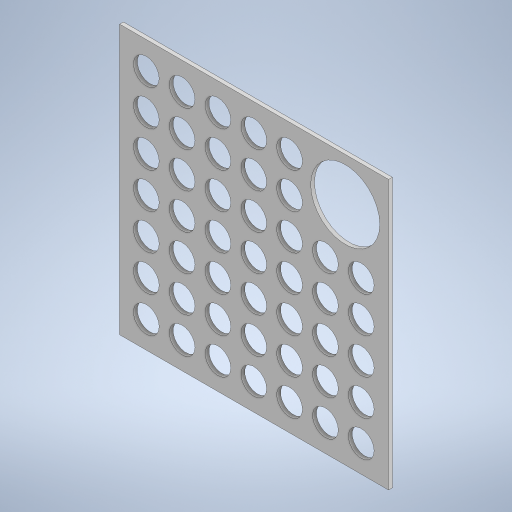
# Autodesk Inventor part: inert indsats plade
Saved by Autodesk Inventor 2023 (Build 270158000, 158)
## iProperties
Created: 2022-10-19
Part Number: inert indsats plade
Material: Generic
Document SubType Name: Modeling
Designer: Jakob Saugbjerg
Density: 1 g/cm^3
Appearance: Default
Author: Jakob Saugbjerg
Autodesk Inventor part; units mm, degrees
ref_plane "YZ Plane" through (0, 0, 0) normal (1, 0, 0) x (0, 1, 0)
ref_plane "XZ Plane" through (0, 0, 0) normal (0, 1, 0) x (-1, 0, 0)
ref_plane "XY Plane" through (0, 0, 0) normal (0, 0, 1) x (1, 0, 0)
sketch "Sketch1" plane through (0, 0, 0) normal (0, 0, 1) x (1, 0, 0)
  line L0 (0, 0) -> (214, 0)
  line L1 (214, 0) -> (214, 214)
  line L2 (214, 214) -> (0, 214)
  line L3 (0, 214) -> (0, 0)
  dimension "d0" = 214
  dimension "d1" = 214
  constraints: 8 end point, 2 parallel, 1 horizontal, 1 perpendicular
  measures "d0" distance of L2.end L1.end
  measures "d1" distance of L1.end L0.end
extrude "Extrusion1" add sketch "Sketch1" along normal blind 3
sketch "Sketch2" plane through (0, 0, 3) normal (0, 0, 1) x (1, 0, 0)
  line L0 (207, 207) -> (7, 207)
  line L1 (7, 207) -> (7, 7)
  line L2 (7, 7) -> (207, 7)
  line L3 (207, 7) -> (207, 207)
  line L4 (207, 207) -> (7, 7) construction
  line L5 (7, 207) -> (207, 7) construction
  line L6 (7, 7) -> (35.5, 7)
  line L7 (35.5, 7) -> (35.5, 35.5)
  line L8 (35.5, 35.5) -> (7, 35.5)
  line L9 (7, 35.5) -> (7, 7)
  circle A0 centre (21.25, 21.25) radius 10.25
  point P0 (0, 0)
  point P1 (107, 107)
  dimension "d4" = 200
  dimension "d5" = 200
  dimension "d6" = 28.5
  dimension "d7" = 28.5
  dimension "d8" = 20.5
  constraints: 20 end point, 4 parallel, 2 horizontal, 2 midpoint, 2 perpendicular, 1 centre point, 1 point on line
  measures "d4" distance of L2.end L1.end
  measures "d5" distance of L1.end L0.end
  measures "d6" distance of L8.end L7.end
  measures "d7" distance of L7.end L6.end
  measures "d8" diameter of A0
extrude "Extrusion2" cut sketch "Sketch2" against normal blind 3 contours A0
pattern_linear "Rectangular Pattern1" count 7 spacing 28.5 along (1, 0, 0) count 5 spacing 28.5 along (0, 1, 0) of "Extrusion2"
sketch "Sketch3" plane through (0, 0, 3) normal (0, 0, 1) x (1, 0, 0)
  circle A0 centre (21.25, 135.25) radius 10.25 projected
  line L0 (21.25, 135.25) -> (21.25, 163.75)
  circle A1 centre (21.25, 163.75) radius 10.25
  point P0 (0, 0)
  dimension "d17" = 28.5
  dimension "d18" = 20.5
  constraints: 2 end point, 1 centre point, 1 coincident, 1 vertical
  measures "d17" distance of L0.start L0.end
  measures "d18" diameter of A1
extrude "Extrusion3" cut sketch "Sketch3" against normal blind 3 contours A1
pattern_linear "Rectangular Pattern2" count 5 spacing 28.5 along (1, 0, 0) count 2 spacing 28.5 along (0, 1, 0) of "Extrusion3"
sketch "Sketch4" plane through (0, 0, 3) normal (0, 0, 1) x (1, 0, 0)
  line L0 (7, 7) -> (207, 7)
  line L1 (207, 7) -> (207, 207)
  line L2 (207, 207) -> (7, 207)
  line L3 (7, 207) -> (7, 7)
  line L4 (7, 7) -> (207, 207) construction
  line L5 (207, 7) -> (7, 207) construction
  line L6 (207, 207) -> (152, 207)
  line L7 (152, 207) -> (152, 152)
  line L8 (152, 152) -> (207, 152)
  line L9 (207, 152) -> (207, 207)
  circle A0 centre (179.5, 179.5) radius 27.5
  point P0 (0, 0)
  point P1 (107, 107)
  dimension "d27" = 200
  dimension "d28" = 200
  dimension "d29" = 55
  dimension "d30" = 55
  constraints: 20 end point, 4 parallel, 2 horizontal, 2 midpoint, 2 perpendicular, 1 centre point, 1 point on line, 1 tangent
  measures "d27" distance of L2.end L1.end
  measures "d28" distance of L1.end L0.end
  measures "d29" distance of L8.end L7.end
  measures "d30" distance of L7.end L6.end
extrude "Extrusion4" cut sketch "Sketch4" against normal blind 3 contours A0
body "Solid1"
